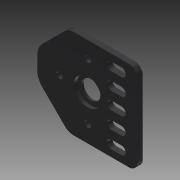
# Autodesk Inventor part: VSLOT Threaded Rod Plate
Saved by Autodesk Inventor 2014 SP1 (Build 180222100, 222)
## iProperties
Created: 2016-04-10
Part Number: VSLOT Threaded Rod Plate
Material: Generic
Document SubType Name: Modeling
Designer: Ben
Density: 1 g/cm^3
Appearance: Default
Author: Ben
Autodesk Inventor part; units mm, degrees
ref_plane "YZ Plane" through (0, 0, 0) normal (1, 0, 0) x (0, 1, 0)
ref_plane "XZ Plane" through (0, 0, 0) normal (0, 1, 0) x (-1, 0, 0)
ref_plane "XY Plane" through (0, 0, 0) normal (0, 0, 1) x (1, 0, 0)
sketch "Sketch1" plane through (0, 0, 0) normal (0, 0, 1) x (1, 0, 0)
  line L0 (-29.86, 26.5) -> (29.43, 26.5)
  line L1 (29.43, 26.5) -> (29.43, -26.5)
  line L2 (29.43, -26.5) -> (-29.86, -26.5)
  line L3 (-29.86, -26.5) -> (-29.86, 26.5)
  line L4 (-29.86, 0) -> (29.43, 0) construction
  circle A0 centre (0, 0) radius 5.5
  dimension "d0" = 29.86
  dimension "d1" = 59.29
  dimension "d2" = 53
  dimension "d3" = 11
  constraints: 10 end point, 2 midpoint, 2 parallel, 1 centre point, 1 coincident, 1 horizontal, 1 perpendicular, 1 point on line
  measures "d0" distance from line of L3 point (0, 0)
  measures "d1" distance of L0.start L0.end
  measures "d2" distance of L0.end L1.end
  measures "d3" diameter of A0
extrude "Extrusion1" add sketch "Sketch1" along normal blind 3.17
sketch "Sketch2" plane through (0, 0, 3.17) normal (0, 0, 1) x (1, 0, 0)
  circle A0 centre (0, 0) radius 5.5 projected
  line L0 (29.43, -26.5) -> (29.43, 26.5) projected
  line L1 (0, 0) -> (0, 49.2966)
  circle A1 centre (0, 16.6681) radius 1.8076
  circle A2 centre (-16.6681, 0) radius 1.8076
  circle A3 centre (0, -16.6681) radius 1.8076
  dimension "d8" = 180
  constraints: 3 centre point, 2 end point, 1 parallel, 1 point on line, 5 other
extrude "Extrusion2" cut sketch "Sketch2" against normal up to next contours A1 L1 | L1 A1 | A2 | A3
sketch "Sketch3" plane through (0, 0, 3.17) normal (0, 0, 1) x (1, 0, 0)
  circle A0 centre (0, 0) radius 5.5 projected
  circle A1 centre (0, 0) radius 8.025
  dimension "d12" = 16.05
  constraints: 1 centre point, 1 coincident
  measures "d12" diameter of A1
extrude "Extrusion3" cut sketch "Sketch3" against normal blind 2
sketch "Sketch4" plane through (0, 0, 3.17) normal (0, 0, 1) x (1, 0, 0)
  line L0 (29.43, 26.5) -> (-29.86, 26.5) projected
  line L1 (-29.86, 26.5) -> (-29.86, -26.5) projected
  line L2 (29.43, -26.5) -> (29.43, 26.5) projected
  line L3 (14, 0) -> (19.9977, 0) construction
  line L4 (14, -2.5) -> (19.9977, -2.5)
  line L5 (19.9977, 2.5) -> (14, 2.5)
  arc A0 (14, 2.5) -> (14, -2.5) centre (14, 0) ccw
  arc A1 (19.9977, -2.5) -> (19.9977, 2.5) centre (19.9977, 0) ccw
  line L6 (14, 10) -> (19.9977, 10) construction
  line L7 (14, 7.5) -> (19.9977, 7.5)
  line L8 (19.9977, 12.5) -> (14, 12.5)
  arc A2 (14, 12.5) -> (14, 7.5) centre (14, 10) ccw
  arc A3 (19.9977, 7.5) -> (19.9977, 12.5) centre (19.9977, 10) ccw
  line L9 (14, 20) -> (19.9977, 20) construction
  line L10 (14, 17.5) -> (19.9977, 17.5)
  line L11 (19.9977, 22.5) -> (14, 22.5)
  arc A4 (14, 22.5) -> (14, 17.5) centre (14, 20) ccw
  arc A5 (19.9977, 17.5) -> (19.9977, 22.5) centre (19.9977, 20) ccw
  line L12 (14, -10) -> (19.9977, -10) construction
  line L13 (14, -12.5) -> (19.9977, -12.5)
  line L14 (19.9977, -7.5) -> (14, -7.5)
  arc A6 (14, -7.5) -> (14, -12.5) centre (14, -10) ccw
  arc A7 (19.9977, -12.5) -> (19.9977, -7.5) centre (19.9977, -10) ccw
  line L15 (14, 0) -> (19.9977, 0) construction
  line L16 (14, -2.5) -> (19.9977, -2.5)
  line L17 (19.9977, 2.5) -> (14, 2.5)
  arc A8 (14, 2.5) -> (14, -2.5) centre (14, 0) ccw
  arc A9 (19.9977, -2.5) -> (19.9977, 2.5) centre (19.9977, 0) ccw
  line L18 (14, 10) -> (19.9977, 10) construction
  line L19 (14, 7.5) -> (19.9977, 7.5)
  line L20 (19.9977, 12.5) -> (14, 12.5)
  arc A10 (14, 12.5) -> (14, 7.5) centre (14, 10) ccw
  arc A11 (19.9977, 7.5) -> (19.9977, 12.5) centre (19.9977, 10) ccw
  line L21 (14, -20) -> (19.9977, -20) construction
  line L22 (14, -22.5) -> (19.9977, -22.5)
  line L23 (19.9977, -17.5) -> (14, -17.5)
  arc A12 (14, -17.5) -> (14, -22.5) centre (14, -20) ccw
  arc A13 (19.9977, -22.5) -> (19.9977, -17.5) centre (19.9977, -20) ccw
  line L24 (14, -10) -> (19.9977, -10) construction
  line L25 (14, -12.5) -> (19.9977, -12.5)
  line L26 (19.9977, -7.5) -> (14, -7.5)
  arc A14 (14, -7.5) -> (14, -12.5) centre (14, -10) ccw
  arc A15 (19.9977, -12.5) -> (19.9977, -7.5) centre (19.9977, -10) ccw
  line L27 (14, 0) -> (19.9977, 0) construction
  line L28 (14, -2.5) -> (19.9977, -2.5)
  line L29 (19.9977, 2.5) -> (14, 2.5)
  arc A16 (14, 2.5) -> (14, -2.5) centre (14, 0) ccw
  arc A17 (19.9977, -2.5) -> (19.9977, 2.5) centre (19.9977, 0) ccw
  point P0 (16.9988, 0)
  point P1 (16.9988, 10)
  point P2 (16.9988, 20)
  point P3 (16.9988, -10)
  point P4 (16.9988, 0)
  point P5 (16.9988, 10)
  point P6 (16.9988, -20)
  point P7 (16.9988, -10)
  point P8 (16.9988, 0)
  dimension "d15" = 5
  dimension "d16" = 43.86
  dimension "d19" = 10
  dimension "d22" = 10
  constraints: 72 end point, 36 point on circle, 18 centre point, 4 tangent, 2 parallel, 2 vertical, 1 midpoint, 96 other
  measures "d15" diameter of A1
  measures "d16" distance from line of L1 L3.start
  measures "d19" distance of L4.start L7.start
  measures "d22" distance of L4.start L13.start
extrude "Extrusion4" cut sketch "Sketch4" against normal up to next
sketch "Sketch5" plane through (0, 0, 3.17) normal (0, 0, 1) x (1, 0, 0)
  line L0 (29.43, 26.5) -> (-29.86, 26.5) projected
  line L1 (-29.86, 26.5) -> (-29.86, -26.5) projected
  line L2 (-29.86, -26.5) -> (29.43, -26.5) projected
  line L3 (-29.86, 8.025) -> (-11.385, 26.5)
  line L4 (-29.86, 8.025) -> (-3.7324, 8.025) construction
  line L5 (-29.86, -8.025) -> (-11.385, -26.5)
  dimension "d27" = 45
  constraints: 6 end point, 4 point on line, 1 equal length, 1 horizontal, 1 perpendicular
  measures "d27" angle of L4 L3
extrude "Extrusion5" cut sketch "Sketch5" against normal up to next
fillet "Fillet1" radius 7.25 2 edges at (-11.385, -26.5, 1.585) (-11.385, 26.5, 1.585)
fillet "Fillet2" radius 10.68 2 edges at (-29.86, -8.025, 1.585) (-29.86, 8.025, 1.585)
fillet "Fillet3" radius 5 2 edges at (29.43, 26.5, 1.585) (29.43, -26.5, 1.585)
body "Solid1"
